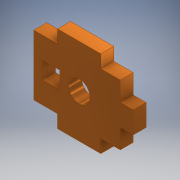
# Autodesk Inventor part: Barilla
Saved by Autodesk Inventor 2018 (Build 220112000, 112)
## iProperties
Created: 2020-03-13
Part Number: Barilla
Material: Oro
Document SubType Name: Modeling
Designer: joser
Density: 19.3 g/cm^3
Appearance: Metal 1600F
Author: joser
Autodesk Inventor part; units mm, degrees
ref_plane "YZ Plane" through (0, 0, 0) normal (1, 0, 0) x (0, 1, 0)
ref_plane "XZ Plane" through (0, 0, 0) normal (0, 1, 0) x (-1, 0, 0)
ref_plane "XY Plane" through (0, 0, 0) normal (0, 0, 1) x (1, 0, 0)
sketch "Boceto1" plane through (0, 0, 0) normal (0, 1, 0) x (-1, 0, 0)
  line L0 (0, 0) -> (-10, 0)
  line L1 (-17.5, -7.5) -> (-17.5, -12.5)
  line L2 (-10, -20) -> (0, -20)
  line L3 (5.5, -17) -> (5.5, -3)
  line L4 (0, -3) -> (0, 0)
  line L5 (-10, -3) -> (-10, 0)
  line L6 (-14.5, -3) -> (-10, -3)
  line L7 (0, -3) -> (5.5, -3)
  line L8 (0, -17) -> (0, -20)
  line L9 (-10, -17) -> (-10, -20)
  line L10 (5.5, -17) -> (0, -17)
  line L11 (-10, -17) -> (-14.5, -17)
  line L12 (-14.5, -12.5) -> (-17.5, -12.5)
  line L13 (-14.5, -7.5) -> (-17.5, -7.5)
  line L14 (-14.5, -17) -> (-14.5, -12.5)
  line L15 (-14.5, -7.5) -> (-14.5, -3)
  circle A0 centre (-5, -10) radius 2.5
  line L16 (-0.5, -8) -> (-0.5, -12)
  line L17 (-0.5, -12) -> (3.5, -12)
  line L18 (3.5, -12) -> (3.5, -8)
  line L19 (3.5, -8) -> (-0.5, -8)
  point P0 (-17.5, -10)
  point P1 (-5, -20)
  point P2 (-0.5, -10)
  dimension "d0" = 23
  dimension "d1" = 20
  dimension "d4" = 10
  dimension "d6" = 5
  dimension "d7" = 3
  dimension "d8" = 3
  dimension "d10" = 5
  dimension "d13" = 7.5
  dimension "d14" = 4
  dimension "d15" = 4
  dimension "d16" = 2
  constraints: 40 end point, 9 parallel, 8 perpendicular, 7 equal length, 4 horizontal, 3 midpoint, 2 horizontal alignment, 1 centre point, 1 coincident, 1 vertical alignment
  measures "d0" distance between parallel lines of L1 L3
  measures "d1" distance between parallel lines of L2 L0
  measures "d4" distance between parallel lines of L5 L4
  measures "d6" distance between parallel lines of L12 L13
  measures "d7" distance between parallel lines of L10 L2
  measures "d8" distance between parallel lines of L15 L1
  measures "d10" diameter of A0
  measures "d13" distance between parallel lines of L5 L1
  measures "d14" distance of L18.end L17.end
  measures "d15" distance between parallel lines of L16 L18
  measures "d16" distance between parallel lines of L3 L18
extrude "Extrusión2" add sketch "Boceto1" along normal blind 3
